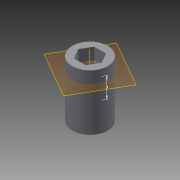
# Autodesk Inventor part: engancheBics
Saved by Autodesk Inventor 2015 SP1 (Build 190203100, 203)
## iProperties
Created: 2015-06-15
Part Number: engancheBics
Material: Genérico
Document SubType Name: Modeling
Designer: Javier
Density: 1 g/cm^3
Appearance: Valor por defecto
Author: Javier
Autodesk Inventor part; units mm, degrees
ref_plane "YZ Plane" through (0, 0, 0) normal (1, 0, 0) x (0, 1, 0)
ref_plane "XZ Plane" through (0, 0, 0) normal (0, 1, 0) x (-1, 0, 0)
ref_plane "XY Plane" through (0, 0, 0) normal (0, 0, 1) x (1, 0, 0)
sketch "Boceto1" plane through (0, 0, 0) normal (0, 0, 1) x (1, 0, 0)
  line L0 (4, 0) -> (2, -3.4641)
  line L1 (2, -3.4641) -> (-2, -3.4641)
  line L2 (-2, -3.4641) -> (-4, 0)
  line L3 (-4, 0) -> (-2, 3.4641)
  line L4 (-2, 3.4641) -> (2, 3.4641)
  line L5 (2, 3.4641) -> (4, 0)
  line L6 (3, 0) -> (1.5, -2.5981)
  line L7 (1.5, -2.5981) -> (-1.5, -2.5981)
  line L8 (-1.5, -2.5981) -> (-3, 0)
  line L9 (-3, 0) -> (-1.5, 2.5981)
  line L10 (-1.5, 2.5981) -> (1.5, 2.5981)
  line L11 (1.5, 2.5981) -> (3, 0)
  circle A0 centre (0, 0) radius 6
  dimension "d0" = 4
  dimension "d1" = 1
  dimension "d2" = 12
  constraints: 24 end point, 3 coincident, 1 centre point, 1 parallel, 26 other
  measures "d0" distance of L3.end L4.end
  measures "d1" distance of L0.start L6.start
  measures "d2" diameter of A0
extrude "Extrusión1" add sketch "Boceto1" along normal blind 7 contours A0
sketch "Boceto2" plane through (0, 0, 7) normal (0, 0, 1) x (1, 0, 0)
  line L0 (2, -3.4641) -> (-2, -3.4641) projected
  line L1 (-2, -3.4641) -> (-4, 0) projected
  line L2 (-4, 0) -> (-2, 3.4641) projected
  line L3 (-2, 3.4641) -> (2, 3.4641) projected
  line L4 (2, 3.4641) -> (4, 0) projected
  line L5 (4, 0) -> (2, -3.4641) projected
  circle A0 centre (0, 0) radius 6 projected
  circle A1 centre (0, 0) radius 3
  circle A2 centre (0, 0) radius 4
  dimension "d5" = 6
  constraints: 2 coincident, 1 centre point, 3 other
  measures "d5" diameter of A1
sketch "Boceto3" plane through (0, 0, 7) normal (0, 0, 1) x (1, 0, 0)
  circle A0 centre (0, 0) radius 3 projected
  circle A1 centre (0, 0) radius 4
  line L0 (2, -3.4641) -> (-2, -3.4641) projected
  line L1 (-2, -3.4641) -> (-4, 0) projected
  line L2 (-4, 0) -> (-2, 3.4641) projected
  line L3 (-2, 3.4641) -> (2, 3.4641) projected
  line L4 (2, 3.4641) -> (4, 0) projected
  line L5 (4, 0) -> (2, -3.4641) projected
  circle A2 centre (0, 0) radius 6 projected
  constraints: 1 coincident, 3 other
extrude "Extrusión2" add sketch "Boceto2" along normal blind 12 contours A2 L0 | L5 A2 | A2 L1 | L4 A2 | A2 L2 | L3 A2 | A0
extrude "Extrusión3" add sketch "Boceto3" along normal blind 1 contours L5 L0 L1 L2 L3 L4
sketch "Boceto4" plane through (2, -3.4641, 8) normal (-0.8660254, 0.5, 0) x (0, 0, 1)
  line L0 (0, 4) -> (7, 4)
  line L1 (0, 4) -> (11, 4) projected
  line L2 (7, 4) -> (7, 0)
  line L3 (0, 0) -> (11, 0) projected
  point P0 (-8, 2)
  dimension "d10" = 7
  constraints: 4 end point, 2 point on line, 1 perpendicular
  measures "d10" distance of L0.start L0.end
ref_plane "Plano de trabajo2" through (4, 0, 15) normal (0, 0, 1) x (-0.5, -0.8660254, 0)
sketch "Boceto5" plane through (4, 0, 15) normal (0, 0, 1) x (-0.5, -0.8660254, 0)
  line L0 (-2, -3.4641) -> (0, 0) projected
  line L1 (6, -3.4641) -> (4, -6.9282) projected
  line L2 (4, -6.9282) -> (0, -6.9282) projected
  line L3 (0, -6.9282) -> (-2, -3.4641) projected
  line L4 (-2, -3.4641) -> (0, 0) projected
  line L5 (0, 0) -> (4, 0) projected
  line L6 (4, 0) -> (6, -3.4641) projected
  point P0 (2, -3.4641)
loft "Solevación1" add profiles "Boceto5" section 1 edges at (-3, 0, 8) section 3 edges at (0, -3.4641, 8) (3, -1.7321, 8) (3, 1.7321, 8) (0, 3.4641, 8) (-3, 1.7321, 8) (-3, -1.7321, 8)
